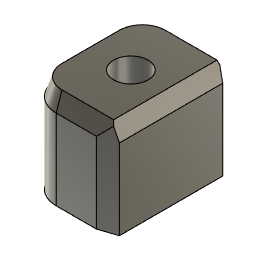
V3D Z Chain Support v4 (Autodesk Fusion 360 design; units mm, degrees)
Autodesk Fusion 360 part; units mm, degrees
note: some values were not read from the file. Chosen so that the rebuilt part matches the saved one: which face or edge a step refers to; which pieces of a blend or face edit are solid.
sketch "Sketch1" plane through (0, 0, 0) normal (0, 1, 0) x (1, 0, 0)
  line L0 (0, 0) -> (0, -17)
  line L1 (0, -17) -> (6, -17)
  line L2 (6, -17) -> (15, -3)
  line L3 (15, -3) -> (15, 0)
  line L4 (15, 0) -> (0, 0)
  line L5 (6, -17) -> (15, -17)
  line L6 (15, -17) -> (15, -3)
  dimension "d1" = 17
  dimension "d2" = 15
  dimension "d3" = 3
  dimension "d4" = 6
  constraint coincident L0.start L4.end
  constraint vertical L0
  constraint perpendicular L0 L1
  constraint perpendicular L1 L3
  constraint perpendicular L0 L4
  constraint parallel L1 L5
  constraint vertical L6
  measures "d1" distance of L0.start L0.end
  measures "d2" distance of L3.end L0.start
  measures "d3" distance of L2.end L3.end
  measures "d4" distance of L0.end L1.end
extrude "Extrude1" add sketch "Sketch1" along normal blind 20
sketch "Sketch2" plane through (0, 0, 0) normal (0, 0, -1) x (1, 0, 0)
  line L0 (15, 0) -> (0, 0)
  line L1 (0, 0) -> (0, -20)
  line L2 (0, -20) -> (15, -20)
  line L3 (15, -20) -> (15, 0)
  circle A0 centre (8, -10) radius 1.75
  circle A1 centre (8, -10) radius 3
  line L4 (0, -10) -> (15, -10) construction
  line L5 (15, -7.1) -> (0, -7.1)
  line L6 (0, -7.1) -> (0, -12.9)
  line L7 (0, -12.9) -> (15, -12.9)
  line L8 (15, -12.9) -> (15, -7.1)
  line L9 (15, -7.1) -> (0, -12.9) construction
  line L10 (0, -7.1) -> (15, -12.9) construction
  point P0 (7.5, -10)
  dimension "d7" = 3.5
  dimension "d8" = 6
  dimension "d12" = 7
  dimension "d17" = 5.8
  constraint concentric A0 A1
  constraint midpoint L1 L4.start
  constraint midpoint L3 L4.end
  constraint coincident A0.centre L4
  constraint horizontal L5
  constraint perpendicular L5 L6
  constraint parallel L5 L7
  constraint parallel L6 L8
  constraint coincident L3 L5.start
  constraint coincident L9 P0
  constraint coincident L10 P0
  constraint midpoint L4 P0
  measures "d7" diameter of A0
  measures "d8" diameter of A1
  measures "d12" distance of L3 A0.centre
  measures "d17" distance of L5 L7
extrude "Extrude4" add sketch "Sketch2" along normal blind 1 contours L3 A1 L5 L7 L8 | L1 A1 L5 L6 L7 | A1 L5 L7
extrude "Extrude2" cut sketch "Sketch2" against normal through all contours A0
extrude "Extrude3" cut sketch "Sketch2" against normal through all from surface at -3 contours A1 L5 | A1 L5 L7 | A1 L7
fillet "Fillet1" radius 5 2 edges at (0, 20, 8.5) (0, 0, 8.5)
chamfer "Chamfer1" distance 1 angle 45 2 edges at (15, 10, -1) (0, 10, -1)
chamfer "Chamfer2" distance 3 distance2 1 7 edges at (1.4645, 1.4645, 17) (10, 0, 17) (10, 20, 17) (1.4645, 18.5355, 17) (0, 10, 17) (15, 0, 8.5) (15, 20, 8.5) measured on face at (0.0057, 4.7621, 5.6667) measured on face at (9.5559, 2.3584, 17) measured on face at (8.3333, 20, 5.6667) measured on face at (0.6699, 17.5, 5.6667) measured on face at (0, 9.0333, 11.3333) measured on face at (15, 9.0333, 11.3333) measured on face at (8.3333, 20, 5.6667)
chamfer "Chamfer3" distance 1.2 angle 45 1 edges at (6.3684, 9.3672, 3)
chamfer "Chamfer4" distance 1 distance2 3 1 edges at (15, 10, 17) measured on face at (9.5559, 3.0251, 17)
